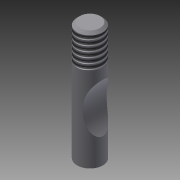
# Autodesk Inventor part: Screwlock
Saved by Autodesk Inventor 2015 (Build 190159000, 159)
## iProperties
Created: 2016-02-24
Part Number: Screwlock
Material: Generic
Document SubType Name: Modeling
Designer: 672301
Density: 1 g/cm^3
Appearance: Default
Author: 672301
Autodesk Inventor part; units mm, degrees
ref_plane "YZ Plane" through (0, 0, 0) normal (1, 0, 0) x (0, 1, 0)
ref_plane "XZ Plane" through (0, 0, 0) normal (0, 1, 0) x (-1, 0, 0)
ref_plane "XY Plane" through (0, 0, 0) normal (0, 0, 1) x (1, 0, 0)
sketch "Sketch1" plane through (0, 0, 0) normal (0, 1, 0) x (-1, 0, 0)
  circle A0 centre (0, 0) radius 1.9685
  dimension "d0" = 3.937
  constraints: 1 centre point, 1 coincident
  measures "d0" diameter of A0
extrude "Extrusion1" add sketch "Sketch1" along normal blind 18.034
sketch "Sketch2" plane through (0, 0, 0) normal (0, 0, 1) x (1, 0, 0)
  line L0 (1.9685, 18.034) -> (-1.9685, 18.034) projected
  line L1 (-1.9685, 0) -> (1.9685, 0) projected
  line L2 (1.9685, 0) -> (6.9469, 0) construction
  line L3 (-1.9685, 0) -> (1.9685, 0) projected
  line L4 (6.9469, 0) -> (6.9469, 7.62) construction
  circle A0 centre (6.9469, 7.62) radius 6.223
  point P0 (0, 0)
  dimension "d3" = 4.9784
  dimension "d4" = 7.62
  dimension "d5" = 12.446
  constraints: 4 end point, 1 centre point, 1 coincident, 1 collinear, 1 vertical
  measures "d3" distance of L1.end L2.end
  measures "d4" distance of L2.end L4.end
  measures "d5" diameter of A0
extrude "Extrusion2" cut sketch "Sketch2" along normal through all both and the other way through all
thread "Thread1" size "8-32 UNC" class "2A" standard "ANSI Unified Screw Threads" length 5.08
chamfer "Chamfer1" distance 0.3969 angle 45 1 edges at (1.9685, 18.034, 0)
body "Solid1"
